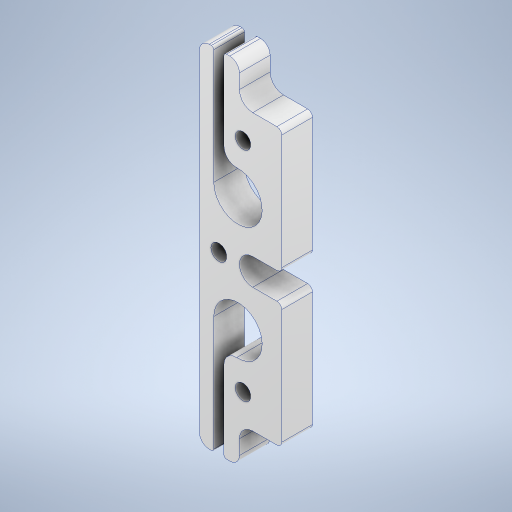
# Autodesk Inventor part: Gantry Belt Clamp
Saved by Autodesk Inventor 2024 (Build 280153000, 153)
## iProperties
Created: 2024-12-26
Part Number: Gantry Belt Clamp
Material: Aluminum 6061
Document SubType Name: Modeling
Designer: Ishaan
Density: 2.7 g/cm^3
Appearance: Aluminum - Flat
Author: Ishaan
Autodesk Inventor part; units mm, degrees
ref_plane "YZ Plane" through (0, 0, 0) normal (1, 0, 0) x (0, 1, 0)
ref_plane "XZ Plane" through (0, 0, 0) normal (0, 1, 0) x (-1, 0, 0)
ref_plane "XY Plane" through (0, 0, 0) normal (0, 0, 1) x (1, 0, 0)
sketch "Sketch1" plane through (0, 0, 0) normal (0, 0, 1) x (1, 0, 0)
  line L0 (8.5, -36.236) -> (-8.5, -36.236)
  line L1 (-8.5, -36.236) -> (-8.5, 36.236)
  line L2 (-8.5, 36.236) -> (8.5, 36.236)
  line L3 (8.5, 36.236) -> (8.5, -36.236)
  line L4 (8.5, -36.236) -> (-8.5, 36.236) construction
  line L5 (-8.5, -36.236) -> (8.5, 36.236) construction
  line L6 (8.5, 0) -> (2.5, 0) construction
  line L7 (8.5, 2.75) -> (2.5, 2.75)
  line L8 (2.5, -2.75) -> (8.5, -2.75)
  arc A0 (8.5, -2.75) -> (8.5, 2.75) centre (8.5, 0) ccw
  arc A1 (2.5, 2.75) -> (2.5, -2.75) centre (2.5, 0) ccw
  line L9 (8.5, 36.236) -> (-0.25, 36.236)
  line L10 (-0.25, 36.236) -> (-0.25, 31.236)
  line L11 (2.5, 28.486) -> (8.5, 28.486)
  line L12 (8.5, 28.486) -> (8.5, 36.236)
  line L13 (8.5, -36.236) -> (-0.25, -36.236)
  line L14 (-0.25, -36.236) -> (-0.25, -31.236)
  line L15 (2.5, -28.486) -> (8.5, -28.486)
  line L16 (8.5, -28.486) -> (8.5, -36.236)
  arc A2 (2.5, -28.486) -> (-0.25, -31.236) centre (2.5, -31.236) ccw
  arc A3 (-0.25, 31.236) -> (2.5, 28.486) centre (2.5, 31.236) ccw
  line L17 (0.5, 22.5) -> (0.5, -22.5) construction
  line L18 (-5.55, 36.236) -> (-3.45, 36.236)
  line L19 (-3.45, 36.236) -> (-3.45, -36.236)
  line L20 (-3.45, -36.236) -> (-5.55, -36.236)
  line L21 (-5.55, -36.236) -> (-5.55, 36.236)
  line L22 (-8.5, 36.236) -> (-0.25, 36.236)
  circle A4 centre (-0.55, 12) radius 3.5
  circle A5 centre (-0.55, 12) radius 5
  circle A6 centre (-0.95, 19.4893) radius 2.5
  circle A7 centre (-4.5, 0) radius 4 construction
  point P0 (0, 0)
  point P1 (5.5, 0)
  point P2 (0.5, 0)
  point P3 (-8.5, 0)
  point P4 (-0.25, -36.236)
  point P5 (8.5, -28.486)
  point P6 (-0.25, 36.236)
  point P7 (-0.8167, 16.9929)
  point P8 (-3.45, 19.4893)
  point P9 (-3.45, 36.236)
  point P10 (-5.55, 36.236)
  point P11 (-5.55, 12)
  dimension "d0" = 17
  dimension "d1" = 72.472
  dimension "d3" = 5.5
  dimension "d4" = 11
  dimension "d6" = 5
  dimension "d7" = 5
  dimension "d8" = 45
  dimension "d9" = 9
  dimension "d22" = 2.1
  dimension "d24" = 7
  dimension "d25" = 1.5
  dimension "d26" = 5
  dimension "d27" = 12
  dimension "d29" = 8
  dimension "d40" = 2.95
  constraints: 48 end point, 12 tangent, 9 parallel, 8 centre point, 8 point on circle, 6 midpoint, 5 perpendicular, 4 horizontal, 3 coincident, 3 collinear, 2 equal radius, 2 horizontal alignment, 2 vertical alignment, 1 vertical
  measures "d0" distance of L1.end L2.end
  measures "d1" distance of L0.end L1.end
  measures "d3" diameter of A1
  measures "d4" distance from line of L1 L6.end
  measures "d6" distance from line of A2.centre L0
  measures "d7" distance from line of L2 A3.centre
  measures "d8" distance of L17.start L17.end
  measures "d9" distance between parallel lines of L17 L1
  measures "d22" distance between parallel lines of L21 L19
  measures "d24" diameter of A4
  measures "d25" radial gap between concentric circles of A4 A5
  measures "d26" diameter of A6
  measures "d27" distance from line of A4.centre L6
  measures "d29" diameter of A7
  measures "d40" distance between parallel lines of L21 L1
extrude "Extrusion1" add sketch "Sketch1" along normal blind 6.35 contours L0 L19 A5 A6 L2 L10 A3 L11 L3 L7 A1 L8 L15 A2 L14 | L0 L21 A5 L19 | L0 L1 L2 L21 | A5 L19 A4 | L19 A4 A5 | L21 L2 L19 A5 | A4 L19 | L19 A4 | L19 A6 A5 | A6
fillet "Fillet1" radius 2 2 edges at (-8.5, -36.236, 3.175) (-8.5, 36.236, 3.175)
fillet "Fillet2" radius 2 2 edges at (-0.25, -36.236, 3.175) (-0.25, 36.236, 3.175)
fillet "Fillet3" radius 1 4 edges at (8.5, -28.486, 3.175) (8.5, -2.75, 3.175) (8.5, 2.75, 3.175) (8.5, 28.486, 3.175)
hole "Hole1" at (0.5, 22.5, 0) at (0.5, -22.5, 0) direction (0, 0, 1) diameter 3.2 end through all
hole "Hole2" at (-4.5, 0, 0) direction (0, 0, 1) diameter 3.3 end through all
extrude "Extrusion2" cut sketch "Sketch1" along normal blind 6.35 contours A5 L19 A4 | L19 A4 A5 | L21 L2 L19 A5 | A4 L19 | L19 A4 | L19 A6 A5
mirror "Mirror1" about plane through (0, 0, 0) normal (0, 1, 0) of "Extrusion2"
fillet "Fillet4" radius 0.5 4 edges at (-5.55, 36.236, 3.175) (-3.45, 36.236, 3.175) (-3.45, -36.236, 3.175) (-5.55, -36.236, 3.175)
equation "\"d7\" = d6"
body "Solid1"
